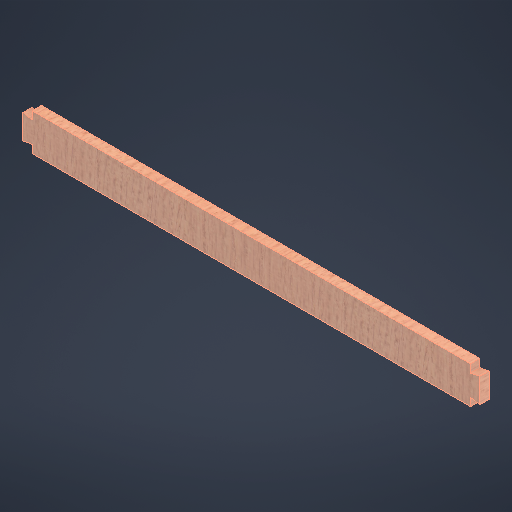
# Autodesk Inventor part: BASE_FRONT,BACK_TREBUCHET
Saved by Autodesk Inventor 2026.2 (Build 302298010, 298A)
## iProperties
Created: 2026-02-18
Part Number: BASE_FRONT,BACK_TREBUCHET
Material: Wood (Oak)
Document SubType Name: Modeling
Designer: 4aida
Density: 0.76 g/cm^3
Appearance: White Oak - Natural Medium Gloss
Author: 4aida
Autodesk Inventor part; units mm, degrees
ref_plane "YZ Plane" through (0, 0, 0) normal (1, 0, 0) x (0, 1, 0)
ref_plane "XZ Plane" through (0, 0, 0) normal (0, 1, 0) x (-1, 0, 0)
ref_plane "XY Plane" through (0, 0, 0) normal (0, 0, 1) x (1, 0, 0)
sketch "Sketch1" plane through (0, 0, 0) normal (0, 0, 1) x (1, 0, 0)
  line L0 (225.425, -19.05) -> (-225.425, -19.05)
  line L1 (-225.425, 19.05) -> (225.425, 19.05)
  line L2 (-225.425, -19.05) -> (225.425, 19.05) construction
  line L3 (-225.425, 10.795) -> (-234.95, 12.7)
  line L4 (-234.95, 12.7) -> (-234.95, -12.7)
  line L5 (-234.95, -12.7) -> (-225.425, -10.795)
  line L6 (-234.95, -12.7) -> (-225.425, -12.7) construction
  line L7 (0, 0) -> (0, 19.05) construction
  line L8 (-225.425, -19.05) -> (-225.425, -10.795)
  line L9 (-225.425, 10.795) -> (-225.425, 19.05)
  line L10 (225.425, 10.795) -> (234.95, 12.7)
  line L11 (234.95, 12.7) -> (234.95, -12.7)
  line L12 (234.95, -12.7) -> (225.425, -10.795)
  line L13 (234.95, -12.7) -> (225.425, -12.7) construction
  line L14 (225.425, -19.05) -> (225.425, -10.795)
  line L15 (225.425, 10.795) -> (225.425, 19.05)
  point P0 (-234.95, 0)
  point P1 (-234.95, 0)
  point P2 (234.95, 0)
  point P3 (234.95, 0)
  dimension "d1" = 9.525
  dimension "d2" = 1.905
  dimension "d3" = 38.1
  dimension "d4" = 25.4
  dimension "d6" = 225.425
  constraints: 32 end point, 7 symmetric about line, 4 perpendicular, 3 coincident, 3 midpoint, 2 equal length, 2 point on line, 2 vertical, 1 horizontal, 1 horizontal alignment, 1 parallel
  measures "d1" distance of L4.end L6.end
  measures "d2" distance from line of L5.end L6
  measures "d3" distance of L0.end L1.start
  measures "d4" distance of L3.end L4.end
  measures "d6" distance from line of L7.start L8
extrude "Extrusion1" add sketch "Sketch1" along normal blind 9.525
equation "\"d2\" = 0.2 * d1"
body "Solid1"
